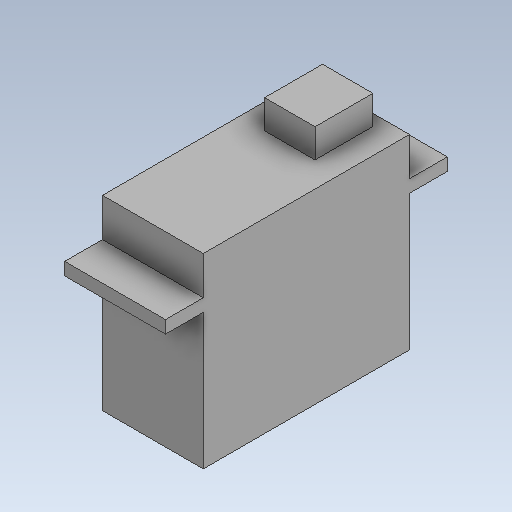
# Autodesk Inventor part: servo
Saved by Autodesk Inventor 2021 (Build 250183000, 183)
## iProperties
Created: 2021-06-15
Part Number: servo
Material: Generic
Document SubType Name: Modeling
Designer: josep
Density: 1 g/cm^3
Appearance: Default
Author: josep
Autodesk Inventor part; units mm, degrees
ref_plane "YZ Plane" through (0, 0, 0) normal (1, 0, 0) x (0, 1, 0)
ref_plane "XZ Plane" through (0, 0, 0) normal (0, 1, 0) x (-1, 0, 0)
ref_plane "XY Plane" through (0, 0, 0) normal (0, 0, 1) x (1, 0, 0)
sketch "Sketch1" plane through (0, 0, 0) normal (1, 0, 0) x (0, 1, 0)
  line L0 (8.7098, 9.3403) -> (-28.2902, 9.3403)
  line L1 (-28.2902, 9.3403) -> (-28.2902, -31.5597)
  line L2 (-28.2902, -31.5597) -> (8.7098, -31.5597)
  line L3 (8.7098, -31.5597) -> (8.7098, 9.3403)
  line L4 (8.7098, -29.3092) -> (14.4098, -29.3092)
  line L5 (14.4098, -29.3092) -> (14.4098, -17.8188)
  line L6 (14.4098, -17.8188) -> (8.7098, -17.8188)
  line L7 (8.7098, -17.8188) -> (8.7098, -29.3092)
  point P0 (0, 0)
  dimension "d0" = 37
  dimension "d1" = 40.9
  dimension "d2" = 5.7
  constraints: 16 end point, 4 parallel, 2 horizontal, 2 perpendicular, 1 point on line
  measures "d0" distance of L2.end L1.end
  measures "d1" distance of L1.end L0.end
  measures "d2" distance of L6.end L5.end
extrude "Extrusion1" add sketch "Sketch1" along normal blind 20
sketch "Sketch2" plane through (20, 0, 0) normal (1, 0, 0) x (0, 0, -1)
  line L0 (29.3092, 14.4098) -> (17.8188, 14.4098) projected
  line L1 (29.3092, 8.7098) -> (29.3092, 14.4098) projected
  line L2 (17.8188, 14.4098) -> (29.3092, 14.4098)
  line L3 (29.3092, 14.4098) -> (29.3092, 8.7098)
  line L4 (29.3092, 8.7098) -> (17.8188, 8.7098)
  line L5 (17.8188, 8.7098) -> (17.8188, 14.4098)
  point P0 (0, 0)
  constraints: 8 end point, 2 parallel, 1 horizontal, 1 perpendicular
extrude "Extrusion2" cut sketch "Sketch2" against normal blind 5
sketch "Sketch3" plane through (0, 0, 0) normal (-1, 0, 0) x (0, 0, 1)
  line L0 (-17.8188, 14.4098) -> (-29.3092, 14.4098) projected
  line L1 (-17.8188, 8.7098) -> (-17.8188, 14.4098) projected
  line L2 (-29.3092, 14.4098) -> (-17.8188, 14.4098)
  line L3 (-17.8188, 14.4098) -> (-17.8188, 8.7098)
  line L4 (-17.8188, 8.7098) -> (-29.3092, 8.7098)
  line L5 (-29.3092, 8.7098) -> (-29.3092, 14.4098)
  point P0 (0, 0)
  constraints: 8 end point, 2 parallel, 1 horizontal, 1 perpendicular
extrude "Extrusion3" cut sketch "Sketch3" against normal blind 5
sketch "Sketch4" plane through (0, 0, 0) normal (-1, 0, 0) x (0, 0, 1)
  line L0 (9.3403, -28.2902) -> (-31.5597, -28.2902) projected
  line L1 (9.3403, -28.2902) -> (9.3403, -1.3902)
  line L2 (9.3403, 8.7098) -> (9.3403, -28.2902) projected
  line L3 (9.3403, -1.3902) -> (16.8403, -1.3902)
  line L4 (16.8403, -1.3902) -> (16.8403, 1.1098)
  line L5 (16.8403, 1.1098) -> (9.3403, 1.1098)
  line L6 (9.3403, 1.1098) -> (9.3403, -1.3902)
  line L7 (-31.5597, -28.2902) -> (-31.5597, 8.7098) projected
  line L8 (-31.5597, -1.3902) -> (-39.0597, -1.3902)
  line L9 (-39.0597, -1.3902) -> (-39.0597, 1.1098)
  line L10 (-39.0597, 1.1098) -> (-31.5597, 1.1098)
  line L11 (-31.5597, 1.1098) -> (-31.5597, -1.3902)
  point P0 (0, 0)
  dimension "d9" = 26.9
  dimension "d10" = 7.5
  dimension "d11" = 2.5
  dimension "d12" = 7.5
  constraints: 18 end point, 3 point on line, 2 horizontal, 2 parallel, 2 perpendicular, 1 collinear, 1 vertical
  measures "d9" distance of L0.start L1.end
  measures "d10" distance of L1.end L3.end
  measures "d11" distance of L3.end L4.end
  measures "d12" distance of L9.end L10.end
extrude "Extrusion4" add sketch "Sketch4" against normal blind 20
body "Solid1"
